# Autodesk Inventor part: Disc Cam
Saved by Autodesk Inventor 2015 (Build 190159000, 159)
## iProperties
Created: 2015-04-14
Part Number: Disc Cam
Material: Stainless Steel, Austenitic
Document SubType Name: Modeling
Designer: WASHHSST
Manufacturer: Standard
Standards Organization: Custom
Density: 1 g/cm^3
Appearance: Steel
CustomPartVersion: 1
Author: WASHHSST
Autodesk Inventor part; units mm, degrees
ref_plane "YZ Plane" through (0, 0, 0) normal (1, 0, 0) x (0, 1, 0)
ref_plane "XZ Plane" through (0, 0, 0) normal (0, 1, 0) x (-1, 0, 0)
ref_plane "XY Plane" through (0, 0, 0) normal (0, 0, 1) x (1, 0, 0)
sketch "Main Sketch" plane through (0, 0, 0) normal (0, 0, 1) x (1, 0, 0)
  spline S0 degree 5 poles (0, 101.6) (2.5604, 101.6) (6.8283, 101.4667) (13.2205, 100.9395) (21.6738, 99.6325) (32.0069, 97.0735) (41.6378, 93.852) (51.2942, 89.7155) (60.5187, 84.8346) (69.2547, 79.2073) (77.4192, 72.8086) (84.9107, 65.5692) (91.6225, 57.4552) (97.4291, 48.4798) (102.2032, 38.7227) (105.8489, 28.2747) (108.2737, 17.3519) (109.5118, 5.9807) (109.4927, -5.3287) (108.0674, -16.775) (105.2944, -28.0052) (101.1814, -38.9158) (95.8029, -49.3021) (89.2461, -59.021) (81.6316, -67.9256) (73.097, -75.9034) (63.7925, -82.8666) (53.8763, -88.7572) (43.4969, -93.5471) (32.8148, -97.2258) (21.9349, -99.8198) (11.0372, -101.3348) (0.0741, -101.8637) (-10.5607, -101.3386) (-21.1722, -99.6545) (-31.4728, -96.896) (-41.4401, -93.0704) (-50.9385, -88.2301) (-59.8833, -82.4217) (-68.1702, -75.7109) (-75.7109, -68.1703) (-82.4218, -59.883) (-88.2298, -50.9395) (-93.071, -41.4379) (-96.8926, -31.4823) (-99.6526, -21.1818) (-101.3208, -10.6492) (-101.8789, 0) (-101.3208, 10.6493) (-99.6527, 21.1818) (-96.8926, 31.4823) (-93.0711, 41.4379) (-88.2298, 50.9395) (-82.4218, 59.8829) (-75.7108, 68.1703) (-68.1703, 75.7108) (-59.883, 82.4218) (-50.9393, 88.2297) (-41.4383, 93.0712) (-31.8798, 96.7395) (-21.5991, 99.5535) (-13.1762, 100.9304) (-6.8111, 101.4671) (-2.5552, 101.6) (0, 101.6) knots 0 0 0 0 0 0 0.019849 0.033064 0.049558 0.066008 0.082403 0.098742 0.115045 0.131342 0.147675 0.164083 0.180604 0.197263 0.214063 0.230973 0.247977 0.26506 0.282204 0.299393 0.316637 0.333919 0.351219 0.368515 0.385787 0.403016 0.420182 0.43727 0.454268 0.47117 0.487952 0.504635 0.521239 0.537784 0.554292 0.570799 0.587307 0.603815 0.620322 0.63683 0.653338 0.669846 0.686353 0.702861 0.719369 0.735876 0.752384 0.768892 0.7854 0.801907 0.818415 0.834923 0.851431 0.867938 0.884446 0.900954 0.917461 0.933969 0.950477 0.966985 0.980191 1 1 1 1 1 1
  point P0 (21.2395, 99.4841)
  point P1 (31.5928, 96.9786)
  point P2 (41.6219, 93.6268)
  point P3 (51.2582, 89.4948)
  point P4 (60.4455, 84.6194)
  point P5 (69.124, 79.0058)
  point P6 (77.2162, 72.6296)
  point P7 (84.6384, 65.4353)
  point P8 (91.2961, 57.3777)
  point P9 (97.0714, 48.4613)
  point P10 (101.8404, 38.7439)
  point P11 (105.4932, 28.3342)
  point P12 (107.9528, 17.3833)
  point P13 (109.1924, 6.0686)
  point P14 (109.1485, -5.2665)
  point P15 (107.7467, -16.632)
  point P16 (104.9835, -27.8482)
  point P17 (100.888, -38.7333)
  point P18 (95.5222, -49.1116)
  point P19 (88.9787, -58.8213)
  point P20 (81.3759, -67.7206)
  point P21 (72.8527, -75.6931)
  point P22 (63.5605, -82.6513)
  point P23 (53.6561, -88.5369)
  point P24 (43.2946, -93.3201)
  point P25 (32.6227, -96.996)
  point P26 (21.7739, -99.5799)
  point P27 (10.8661, -101.1018)
  point P28 (0, -101.6)
  point P29 (-10.6201, -101.0434)
  point P30 (-21.1238, -99.3798)
  point P31 (-31.3961, -96.6273)
  point P32 (-41.3244, -92.8162)
  point P33 (-50.8, -87.9882)
  point P34 (-59.719, -82.1961)
  point P35 (-67.9837, -75.5035)
  point P36 (-75.5035, -67.9837)
  point P37 (-82.1961, -59.719)
  point P38 (-87.9882, -50.8)
  point P39 (-92.8162, -41.3244)
  point P40 (-96.6273, -31.3961)
  point P41 (-99.3798, -21.1238)
  point P42 (-101.0434, -10.6201)
  point P43 (-101.6, 0)
  point P44 (-101.0434, 10.6201)
  point P45 (-99.3798, 21.1238)
  point P46 (-96.6273, 31.3961)
  point P47 (-92.8162, 41.3244)
  point P48 (-87.9882, 50.8)
  point P49 (-82.1961, 59.719)
  point P50 (-75.5035, 67.9837)
  point P51 (-67.9837, 75.5035)
  point P52 (-59.719, 82.1961)
  point P53 (-50.8, 87.9882)
  point P54 (-41.3244, 92.8162)
  point P55 (-31.3961, 96.6273)
  point P56 (-21.1238, 99.3798)
  point P57 (-10.6201, 101.0434)
  constraints: 60 other
extrude "Cam" add sketch "Main Sketch" along normal blind 12.7
body "Solid1"
